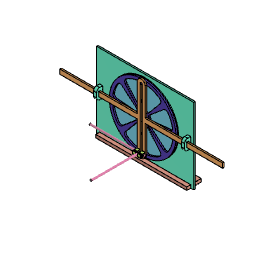
scotchYoke3D (Autodesk Fusion 360 design; units mm, degrees)
Autodesk Fusion 360 part; units mm, degrees
(part 1 of 2)
sketch "Sketch1" plane through (0, 0, 0) normal (0, 1, 0) x (1, 0, 0) in component "Wheel"
  circle A0 centre (0, 0) radius 110
  circle A1 centre (0, -100) radius 3
  line L0 (0, 0) -> (100, 0) construction
  line L1 (2.3568, -26.9387) -> (7.7954, -89.1024)
  arc A2 (6.0037, -21.6842) -> (11.0878, -19.5783) centre (0, 0) ccw
  line L2 (17.382, -20.7151) -> (57.4927, -68.5171)
  line L3 (20.7151, -17.382) -> (68.5171, -57.4927)
  line L4 (26.9387, -2.3568) -> (89.1024, -7.7954)
  arc A3 (12.5, 0) -> (1.0894, -12.4524) centre (0, 0) ccw
  arc A4 (1.0894, -12.4524) -> (8.0348, -9.5756) centre (0, 0) ccw
  arc A5 (8.0348, -9.5756) -> (9.5756, -8.0348) centre (0, 0) ccw
  arc A6 (12.4524, -1.0894) -> (12.5, 0) centre (0, 0) ccw
  arc A7 (9.5756, -8.0348) -> (12.4524, -1.0894) centre (0, 0) ccw
  arc A8 (19.7304, -98.0342) -> (55.3691, -83.2722) centre (0, 0) ccw
  arc A9 (83.2722, -55.3691) -> (98.0342, -19.7304) centre (0, 0) ccw
  arc A10 (7.7954, -89.1024) -> (19.7304, -98.0342) centre (17.7574, -88.2308) ccw
  arc A11 (55.3691, -83.2722) -> (57.4927, -68.5171) centre (49.8322, -74.945) ccw
  arc A12 (6.0037, -21.6842) -> (2.3568, -26.9387) centre (7.3378, -26.503) ccw
  arc A13 (17.382, -20.7151) -> (11.0878, -19.5783) centre (13.5518, -23.929) ccw
  arc A14 (19.5783, -11.0878) -> (20.7151, -17.382) centre (23.929, -13.5518) ccw
  arc A15 (26.9387, -2.3568) -> (21.6842, -6.0037) centre (26.503, -7.3378) ccw
  arc A16 (68.5171, -57.4927) -> (83.2722, -55.3691) centre (74.945, -49.8322) ccw
  arc A17 (98.0342, -19.7304) -> (89.1024, -7.7954) centre (88.2308, -17.7574) ccw
  arc A18 (19.7304, 98.0342) -> (7.7954, 89.1024) centre (17.7574, 88.2308) ccw
  line L5 (2.3568, 26.9387) -> (7.7954, 89.1024)
  arc A19 (2.3568, 26.9387) -> (6.0037, 21.6842) centre (7.3378, 26.503) ccw
  arc A20 (11.0878, 19.5783) -> (6.0037, 21.6842) centre (0, 0) ccw
  arc A21 (11.0878, 19.5783) -> (17.382, 20.7151) centre (13.5518, 23.929) ccw
  line L6 (17.382, 20.7151) -> (57.4927, 68.5171)
  arc A22 (57.4927, 68.5171) -> (55.3691, 83.2722) centre (49.8322, 74.945) ccw
  arc A23 (55.3691, 83.2722) -> (19.7304, 98.0342) centre (0, 0) ccw
  line L7 (20.7151, 17.382) -> (68.5171, 57.4927)
  arc A24 (83.2722, 55.3691) -> (68.5171, 57.4927) centre (74.945, 49.8322) ccw
  arc A25 (98.0342, 19.7304) -> (83.2722, 55.3691) centre (0, 0) ccw
  arc A26 (89.1024, 7.7954) -> (98.0342, 19.7304) centre (88.2308, 17.7574) ccw
  line L8 (26.9387, 2.3568) -> (89.1024, 7.7954)
  arc A27 (21.6842, 6.0037) -> (26.9387, 2.3568) centre (26.503, 7.3378) ccw
  arc A28 (21.6842, 6.0037) -> (19.5783, 11.0878) centre (0, 0) ccw
  arc A29 (20.7151, 17.382) -> (19.5783, 11.0878) centre (23.929, 13.5518) ccw
  line L9 (0, -1.75) -> (0, -22.5) construction
  arc A30 (-11.0878, -19.5783) -> (-6.0037, -21.6842) centre (0, 0) ccw
  arc A31 (-2.3568, -26.9387) -> (-6.0037, -21.6842) centre (-7.3378, -26.503) ccw
  line L10 (-2.3568, -26.9387) -> (-7.7954, -89.1024)
  line L11 (-17.382, -20.7151) -> (-57.4927, -68.5171)
  arc A32 (-19.7304, -98.0342) -> (-7.7954, -89.1024) centre (-17.7574, -88.2308) ccw
  arc A33 (-55.3691, -83.2722) -> (-19.7304, -98.0342) centre (0, 0) ccw
  arc A34 (-57.4927, -68.5171) -> (-55.3691, -83.2722) centre (-49.8322, -74.945) ccw
  arc A35 (-11.0878, -19.5783) -> (-17.382, -20.7151) centre (-13.5518, -23.929) ccw
  arc A36 (-83.2722, -55.3691) -> (-68.5171, -57.4927) centre (-74.945, -49.8322) ccw
  arc A37 (-98.0342, -19.7304) -> (-83.2722, -55.3691) centre (0, 0) ccw
  arc A38 (-89.1024, -7.7954) -> (-98.0342, -19.7304) centre (-88.2308, -17.7574) ccw
  line L12 (-26.9387, -2.3568) -> (-89.1024, -7.7954)
  arc A39 (-21.6842, -6.0037) -> (-26.9387, -2.3568) centre (-26.503, -7.3378) ccw
  arc A40 (-21.6842, -6.0037) -> (-19.5783, -11.0878) centre (0, 0) ccw
  arc A41 (-20.7151, -17.382) -> (-19.5783, -11.0878) centre (-23.929, -13.5518) ccw
  line L13 (-20.7151, -17.382) -> (-68.5171, -57.4927)
  line L14 (-20.7151, 17.382) -> (-68.5171, 57.4927)
  arc A42 (-19.5783, 11.0878) -> (-20.7151, 17.382) centre (-23.929, 13.5518) ccw
  arc A43 (-26.9387, 2.3568) -> (-21.6842, 6.0037) centre (-26.503, 7.3378) ccw
  line L15 (-26.9387, 2.3568) -> (-89.1024, 7.7954)
  arc A44 (-98.0342, 19.7304) -> (-89.1024, 7.7954) centre (-88.2308, 17.7574) ccw
  arc A45 (-83.2722, 55.3691) -> (-98.0342, 19.7304) centre (0, 0) ccw
  arc A46 (-68.5171, 57.4927) -> (-83.2722, 55.3691) centre (-74.945, 49.8322) ccw
  arc A47 (-6.0037, 21.6842) -> (-2.3568, 26.9387) centre (-7.3378, 26.503) ccw
  arc A48 (-17.382, 20.7151) -> (-11.0878, 19.5783) centre (-13.5518, 23.929) ccw
  line L16 (-17.382, 20.7151) -> (-57.4927, 68.5171)
  line L17 (-2.3568, 26.9387) -> (-7.7954, 89.1024)
  arc A49 (-7.7954, 89.1024) -> (-19.7304, 98.0342) centre (-17.7574, 88.2308) ccw
  arc A50 (-19.7304, 98.0342) -> (-55.3691, 83.2722) centre (0, 0) ccw
  arc A51 (-55.3691, 83.2722) -> (-57.4927, 68.5171) centre (-49.8322, 74.945) ccw
  arc A52 (19.5783, -11.0878) -> (21.6842, -6.0037) centre (0, 0) ccw
  arc A53 (-19.5783, 11.0878) -> (-21.6842, 6.0037) centre (0, 0) ccw
  arc A54 (-6.0037, 21.6842) -> (-11.0878, 19.5783) centre (0, 0) ccw
  dimension "d5" = 6
  dimension "d11" = 10
  dimension "d12" = 10
  dimension "d13" = 5
  dimension "d14" = 5
  dimension "d15" = 5
  dimension "d16" = 5
  dimension "d17" = 10
  dimension "d18" = 10
  constraint coincident A0.centre L0.start
  constraint horizontal L0
  constraint concentric A3 A5
  constraint concentric A4 A5
  constraint concentric A5 A6
  constraint concentric A5 A7
  constraint tangent L1 A10
  constraint tangent A8 A10
  constraint tangent L2 A11
  constraint tangent A8 A11
  constraint tangent L1 A12
  constraint tangent A2 A12
  constraint tangent L2 A13
  constraint tangent A2 A13
  constraint tangent L3 A14
  constraint tangent L4 A15
  constraint tangent L3 A16
  constraint tangent A9 A16
  constraint tangent L4 A17
  constraint tangent A9 A17
  constraint symmetric A2 L9 A30
  constraint symmetric A8 L9 A33
  constraint symmetric A9 L9 A37
  constraint symmetric L1.end L9 L10.end
  constraint symmetric A8.start L9 A32.start
  constraint symmetric A10 L9 A32
  constraint symmetric L2.end L9 L11.end
  constraint symmetric A8.end L9 A33.start
  constraint symmetric A11 L9 A34
  constraint symmetric L1.start L9 A31.start
  constraint symmetric A2.start L9 A30.end
  constraint symmetric A12 L9 A31
  constraint symmetric L2.start L9 L11.start
  constraint symmetric A2.end L9 A30.start
  constraint symmetric A13 L9 A35
  constraint symmetric L3.start L9 A41.start
  constraint symmetric A14.start L9 A40.end
  constraint symmetric A14 L9 A41
  constraint symmetric L4.start L9 L12.start
  constraint symmetric A15.end L9 A39.start
  constraint symmetric A15 L9 A39
  constraint symmetric L3.end L9 A36.end
  constraint symmetric A9.start L9 A36.start
  constraint symmetric A16 L9 A36
  constraint symmetric L4.end L9 A38.start
  constraint symmetric A9.end L9 A37.start
  constraint symmetric A17 L9 A38
  constraint symmetric A18.end L9 L17.end
  constraint symmetric A18.start L9 A49.end
  constraint symmetric A18 L9 A49
  constraint symmetric L5.start L9 A47.end
  constraint symmetric A19.end L9 A47.start
  constraint symmetric A19 L9 A47
  constraint symmetric A20.start L9 A48.end
  constraint symmetric A21.end L9 A48.start
  constraint symmetric A21 L9 A48
  constraint symmetric L6.end L9 L16.end
  constraint symmetric A22.end L9 A50.end
  constraint symmetric A22 L9 A51
  constraint symmetric A23 L9 A50
  constraint symmetric L7.start L9 L14.start
  constraint symmetric L7.end L9 L14.end
  constraint symmetric A24.start L9 A45.start
  constraint symmetric A24 L9 A46
  constraint symmetric A25.start L9 A44.start
  constraint symmetric A25 L9 A45
  constraint symmetric A26.start L9 L15.end
  constraint symmetric A26 L9 A44
  constraint symmetric L8.start L9 A43.start
  constraint symmetric A27.start L9 A43.end
  constraint symmetric A27 L9 A43
  constraint symmetric A28.end L9 A42.start
  constraint symmetric A29 L9 A42
  constraint symmetric L9 A39.start A15.end
  constraint symmetric L9 A40.end A14.start
  constraint symmetric L9 A40 A52
  measures "d5" diameter of A1
  measures "d11" radius of A10
  measures "d12" radius of A11
  measures "d13" radius of A12
  measures "d14" radius of A13
  measures "d15" radius of A14
  measures "d16" radius of A15
  measures "d17" radius of A16
  measures "d18" radius of A17
extrude "Extrude1" add sketch "Sketch1" along normal blind 5 contours A0 | A1 makes body 1 in component "Wheel"
extrude "Extrude2" add sketch "Sketch1" against normal blind 5.25 contours A1 bodies 1 in component "Wheel"
extrude "Extrude1'" add sketch "Sketch1" along normal blind 3 separate body contours A0 | A1 | L1 A2 L2 A8 A10 A11 A12 A13 | L3 L4 A9 A14 A15 A16 A17 A52 | A3 A4 A5 A6 A7 | A18 L5 A19 A20 A21 L6 A22 A23 | L7 A24 A25 A26 L8 A27 A28 A29 | A30 A31 L10 L11 A32 A33 A34 A35 | A36 A37 A38 L12 A39 A40 A41 L13 | L14 A42 A43 L15 A44 A45 A46 A53 | A47 A48 L16 L17 A49 A50 A51 A54 makes body 2 in component "BackWheel"
sketch "Sketch1 (2)" plane through (0, 0, 0) normal (0, -1, 0) x (1, 0, 0) in component "Slider"
  circle A0 centre (0, 100) radius 3
  arc A1 (26.9387, -2.3568) -> (21.6842, -6.0037) centre (26.503, -7.3378) ccw
  line L0 (26.9387, -2.3568) -> (89.1024, -7.7954)
  arc A2 (98.0342, -19.7304) -> (89.1024, -7.7954) centre (88.2308, -17.7574) ccw
  arc A3 (83.2722, -55.3691) -> (98.0342, -19.7304) centre (0, 0) ccw
  arc A4 (68.5171, -57.4927) -> (83.2722, -55.3691) centre (74.945, -49.8322) ccw
  line L1 (68.5171, -57.4927) -> (20.7151, -17.382)
  arc A5 (19.5783, -11.0878) -> (20.7151, -17.382) centre (23.929, -13.5518) ccw
  arc A6 (19.5783, -11.0878) -> (21.6842, -6.0037) centre (0, 0) ccw
  arc A7 (17.382, -20.7151) -> (11.0878, -19.5783) centre (13.5518, -23.929) ccw
  line L2 (17.382, -20.7151) -> (57.4927, -68.5171)
  arc A8 (55.3691, -83.2722) -> (57.4927, -68.5171) centre (49.8322, -74.945) ccw
  arc A9 (19.7304, -98.0342) -> (55.3691, -83.2722) centre (0, 0) ccw
  arc A10 (7.7954, -89.1024) -> (19.7304, -98.0342) centre (17.7574, -88.2308) ccw
  line L3 (7.7954, -89.1024) -> (2.3568, -26.9387)
  arc A11 (6.0037, -21.6842) -> (2.3568, -26.9387) centre (7.3378, -26.503) ccw
  arc A12 (6.0037, -21.6842) -> (11.0878, -19.5783) centre (0, 0) ccw
  circle A13 centre (0, 0) radius 12.5
  arc A14 (2.3568, 26.9387) -> (6.0037, 21.6842) centre (7.3378, 26.503) ccw
  line L4 (2.3568, 26.9387) -> (7.7954, 89.1024)
  arc A15 (19.7304, 98.0342) -> (7.7954, 89.1024) centre (17.7574, 88.2308) ccw
  arc A16 (55.3691, 83.2722) -> (19.7304, 98.0342) centre (0, 0) ccw
  arc A17 (57.4927, 68.5171) -> (55.3691, 83.2722) centre (49.8322, 74.945) ccw
  line L5 (57.4927, 68.5171) -> (17.382, 20.7151)
  arc A18 (11.0878, 19.5783) -> (17.382, 20.7151) centre (13.5518, 23.929) ccw
  arc A19 (11.0878, 19.5783) -> (6.0037, 21.6842) centre (0, 0) ccw
  line L6 (20.7151, 17.382) -> (68.5171, 57.4927)
  arc A20 (83.2722, 55.3691) -> (68.5171, 57.4927) centre (74.945, 49.8322) ccw
  arc A21 (98.0342, 19.7304) -> (83.2722, 55.3691) centre (0, 0) ccw
  arc A22 (89.1024, 7.7954) -> (98.0342, 19.7304) centre (88.2308, 17.7574) ccw
  line L7 (89.1024, 7.7954) -> (26.9387, 2.3568)
  arc A23 (21.6842, 6.0037) -> (26.9387, 2.3568) centre (26.503, 7.3378) ccw
  arc A24 (21.6842, 6.0037) -> (19.5783, 11.0878) centre (0, 0) ccw
  arc A25 (20.7151, 17.382) -> (19.5783, 11.0878) centre (23.929, 13.5518) ccw
  arc A26 (-26.9387, 2.3568) -> (-21.6842, 6.0037) centre (-26.503, 7.3378) ccw
  line L8 (-26.9387, 2.3568) -> (-89.1024, 7.7954)
  arc A27 (-98.0342, 19.7304) -> (-89.1024, 7.7954) centre (-88.2308, 17.7574) ccw
  arc A28 (-83.2722, 55.3691) -> (-98.0342, 19.7304) centre (0, 0) ccw
  arc A29 (-68.5171, 57.4927) -> (-83.2722, 55.3691) centre (-74.945, 49.8322) ccw
  line L9 (-68.5171, 57.4927) -> (-20.7151, 17.382)
  arc A30 (-19.5783, 11.0878) -> (-20.7151, 17.382) centre (-23.929, 13.5518) ccw
  arc A31 (-19.5783, 11.0878) -> (-21.6842, 6.0037) centre (0, 0) ccw
  line L10 (-2.3568, -26.9387) -> (-7.7954, -89.1024)
  arc A32 (-19.7304, -98.0342) -> (-7.7954, -89.1024) centre (-17.7574, -88.2308) ccw
  arc A33 (-55.3691, -83.2722) -> (-19.7304, -98.0342) centre (0, 0) ccw
  arc A34 (-57.4927, -68.5171) -> (-55.3691, -83.2722) centre (-49.8322, -74.945) ccw
  line L11 (-57.4927, -68.5171) -> (-17.382, -20.7151)
  arc A35 (-11.0878, -19.5783) -> (-17.382, -20.7151) centre (-13.5518, -23.929) ccw
  arc A36 (-11.0878, -19.5783) -> (-6.0037, -21.6842) centre (0, 0) ccw
  arc A37 (-2.3568, -26.9387) -> (-6.0037, -21.6842) centre (-7.3378, -26.503) ccw
  arc A38 (-6.0037, 21.6842) -> (-2.3568, 26.9387) centre (-7.3378, 26.503) ccw
  arc A39 (-6.0037, 21.6842) -> (-11.0878, 19.5783) centre (0, 0) ccw
  arc A40 (-17.382, 20.7151) -> (-11.0878, 19.5783) centre (-13.5518, 23.929) ccw
  line L12 (-17.382, 20.7151) -> (-57.4927, 68.5171)
  arc A41 (-55.3691, 83.2722) -> (-57.4927, 68.5171) centre (-49.8322, 74.945) ccw
  arc A42 (-19.7304, 98.0342) -> (-55.3691, 83.2722) centre (0, 0) ccw
  arc A43 (-7.7954, 89.1024) -> (-19.7304, 98.0342) centre (-17.7574, 88.2308) ccw
  line L13 (-7.7954, 89.1024) -> (-2.3568, 26.9387)
  line L14 (-20.7151, -17.382) -> (-68.5171, -57.4927)
  arc A44 (-83.2722, -55.3691) -> (-68.5171, -57.4927) centre (-74.945, -49.8322) ccw
  arc A45 (-98.0342, -19.7304) -> (-83.2722, -55.3691) centre (0, 0) ccw
  arc A46 (-89.1024, -7.7954) -> (-98.0342, -19.7304) centre (-88.2308, -17.7574) ccw
  line L15 (-89.1024, -7.7954) -> (-26.9387, -2.3568)
  arc A47 (-21.6842, -6.0037) -> (-26.9387, -2.3568) centre (-26.503, -7.3378) ccw
  arc A48 (-21.6842, -6.0037) -> (-19.5783, -11.0878) centre (0, 0) ccw
  arc A49 (-20.7151, -17.382) -> (-19.5783, -11.0878) centre (-23.929, -13.5518) ccw
  circle A50 centre (0, 0) radius 110
  line L16 (3.25, -100) -> (3.25, 100)
  arc A51 (3.25, 100) -> (-3.25, 100) centre (0, 100) ccw
  line L17 (-3.25, 100) -> (-3.25, -100)
  arc A52 (-3.25, -100) -> (3.25, -100) centre (0, -100) ccw
  line L18 (0, -100) -> (0, 100) construction
  line L19 (-13.25, 100) -> (-13.25, -100)
  arc A53 (-13.25, -100) -> (13.25, -100) centre (0, -100) ccw
  line L20 (13.25, -100) -> (13.25, 100)
  arc A54 (13.25, 100) -> (-13.25, 100) centre (0, 100) ccw
  dimension "d25" = 6.5
  dimension "d26" = 10
  constraint tangent L16 A51
  constraint tangent A51 L17
  constraint parallel L16 L17
  constraint tangent L17 A52
  constraint tangent L16 A52
  constraint coincident A0.centre A51.centre
  constraint vertical L18
  constraint coincident A3.centre A6.centre
  constraint midpoint L18 A3.centre
  measures "d25" diameter of A51
extrude "Extrude1''" add sketch "Sketch1 (2)" along normal blind 5 separate body contours A7 A10 L3 A11 A12 L16 L20 | A7 A11 A12 A13 A14 A18 A19 L16 L20 | A10 L3 L10 A32 A50 L16 L17 A52 L19 A53 L20 | A14 L4 A15 A18 A19 L16 L20 | L4 A15 A43 L13 A50 L16 A51 L17 L19 L20 A54 | A50 A53 | A13 L16 | A50 A54 | A13 A35 A36 A37 A38 A39 A40 L17 L19 | A13 L17 | L10 A32 A35 A36 A37 L17 L19 | A38 A39 A40 A43 L13 L17 L19 makes body 3 in component "Slider"
sketch "Sketch2" plane through (13.25, 0, 0) normal (1, 0, 0) x (0, 1, 0) in component "Slider"
  line L0 (0, -100) -> (0, 100)
  line L1 (0, 100) -> (-5, 100)
  line L2 (-5, 100) -> (-5, -100)
  line L3 (-5, -100) -> (0, -100)
  line L4 (0, 0) -> (-5, 0) construction
  line L5 (0, 7.5) -> (-5, 7.5)
  line L6 (-5, 7.5) -> (-5, -7.5)
  line L7 (-5, -7.5) -> (0, -7.5)
  line L8 (0, -7.5) -> (0, 7.5)
  line L9 (0, 7.5) -> (-5, -7.5) construction
  line L10 (-5, 7.5) -> (0, -7.5) construction
  point P0 (-2.5, 0)
  dimension "d29" = 15
  constraint coincident L4.start origin
  constraint midpoint L2 L4.end
  constraint horizontal L5
  constraint perpendicular L5 L6
  constraint parallel L5 L7
  constraint parallel L6 L8
  constraint coincident L9 P0
  constraint coincident L10 P0
  constraint midpoint L4 P0
  measures "d29" distance of L5.end L6.end
extrude "Extrude2'" add sketch "Sketch2" along normal blind 255 contours L0 L2 L5 L6 L7 L8 bodies 3 in component "Slider"
mirror "Mirror1" about plane through (0, 0, 0) normal (1, 0, 0) of "Extrude2'" in component "Slider"
sketch "Sketch1 (3)" plane through (0, 8, 0) normal (0, 1, 0) x (-1, 0, 0) in component "Board"
  circle A0 centre (0, 0) radius 110
  line L0 (-120, 120) -> (120, 120) construction
  line L1 (120, 120) -> (120, -120) construction
  line L2 (120, -120) -> (-120, -120) construction
  line L3 (-120, -120) -> (-120, 120) construction
  line L4 (-120, 120) -> (120, -120) construction
  line L5 (120, 120) -> (-120, -120) construction
  line L6 (120, 0) -> (130, 0) construction
  line L7 (-120, 0) -> (-130, 0) construction
  line L8 (0, -120) -> (0, -130) construction
  circle A1 centre (0, 0) radius 12.5
  line L9 (0, 0) -> (-150, 0) construction
  line L10 (0, 0) -> (150, 0) construction
  line L11 (150, -130) -> (160, -130) construction
  line L12 (-150, -130) -> (-160, -130) construction
  line L13 (-150, 120) -> (-160, 120) construction
  line L14 (150, 120) -> (160, 120) construction
  line L15 (160, -130) -> (-160, -130)
  line L16 (-160, -130) -> (-160, 120)
  line L17 (-160, 120) -> (160, 120)
  line L18 (160, 120) -> (160, -130)
  dimension "d34" = 240
  dimension "d35" = 240
  dimension "d39" = 25
  dimension "d72" = 150
  dimension "d255" = 10
  dimension "d256" = 10
  dimension "d257" = 10
  dimension "d258" = 10
  constraint horizontal L0
  constraint perpendicular L0 L1
  constraint parallel L0 L2
  constraint parallel L1 L3
  constraint coincident L4 A0.centre
  constraint coincident L5 A0.centre
  constraint coincident A0.centre A1.centre
  constraint midpoint L1 L6.start
  constraint perpendicular L1 L6
  constraint midpoint L3 L7.start
  constraint perpendicular L3 L7
  constraint midpoint L2 L8.start
  constraint perpendicular L2 L8
  constraint horizontal L9
  constraint horizontal L15
  constraint vertical L16
  constraint horizontal L17
  constraint vertical L18
  measures "d34" distance of L1.end L2.end
  measures "d35" distance of L0.end L1.end
  measures "d39" diameter of A1
  measures "d72" distance of A0.centre L9.end
  measures "d255" distance of L11.start L11.end
  measures "d256" distance of L12.start L12.end
  measures "d257" distance of L13.start L13.end
  measures "d258" distance of L14.start L14.end
extrude "Extrude1'''" add sketch "Sketch1 (3)" along normal blind 5 separate body contours A0 | L15 L16 L17 L18 makes body 4 in component "Board"
sketch "Sketch2 (2)" plane through (0, 8, 0) normal (0, -1, 0) x (1, 0, 0) in component "Board"
  circle A0 centre (0, 0) radius 12.5
  line L0 (-130, -130) -> (130, -130) construction
  line L1 (-120, -130) -> (-80, -130)
  line L2 (-80, -130) -> (-80, -120)
  line L3 (-80, -120) -> (-120, -120)
  line L4 (-120, -120) -> (-120, -130)
  line L5 (-70, -130) -> (-30, -130)
  line L6 (-30, -130) -> (-30, -120)
  line L7 (-30, -120) -> (-70, -120)
  line L8 (-70, -120) -> (-70, -130)
  line L9 (-20, -130) -> (20, -130)
  line L10 (20, -130) -> (20, -120)
  line L11 (20, -120) -> (-20, -120)
  line L12 (-20, -120) -> (-20, -130)
  line L13 (30, -130) -> (70, -130)
  line L14 (70, -130) -> (70, -120)
  line L15 (70, -120) -> (30, -120)
  line L16 (30, -120) -> (30, -130)
  line L17 (80, -130) -> (120, -130)
  line L18 (120, -130) -> (120, -120)
  line L19 (120, -120) -> (80, -120)
  line L20 (80, -120) -> (80, -130)
  line L21 (130, -130) -> (150, -130)
  line L22 (150, -130) -> (150, -120)
  line L23 (150, -120) -> (130, -120)
  line L24 (130, -120) -> (130, -130)
  line L25 (-130, -130) -> (-150, -130)
  line L26 (-150, -130) -> (-150, -120)
  line L27 (-150, -120) -> (-130, -120)
  line L28 (-130, -120) -> (-130, -130)
  line L29 (160, 120) -> (-160, 120)
  line L30 (-160, 120) -> (-160, -130)
  line L31 (-160, -130) -> (160, -130)
  line L32 (160, -130) -> (160, 120)
  dimension "d42" = 40
  dimension "d43" = 10
  dimension "d45" = 40
  dimension "d46" = 10
  dimension "d47" = 10
  dimension "d48" = 40
  dimension "d49" = 10
  dimension "d50" = 40
  dimension "d51" = 10
  dimension "d52" = 10
  dimension "d53" = 40
  dimension "d54" = 10
  dimension "d55" = 10
  constraint horizontal L1
  constraint vertical L2
  constraint horizontal L3
  constraint vertical L4
  constraint coincident L0 L1.start
  constraint horizontal L5
  constraint vertical L6
  constraint horizontal L7
  constraint vertical L8
  constraint coincident L0 L5.start
  constraint horizontal L9
  constraint vertical L10
  constraint horizontal L11
  constraint vertical L12
  constraint coincident L0 L9.start
  constraint horizontal L13
  constraint vertical L14
  constraint horizontal L15
  constraint vertical L16
  constraint coincident L0 L13.start
  constraint horizontal L17
  constraint vertical L18
  constraint horizontal L19
  constraint vertical L20
  constraint coincident L0 L17.start
  constraint horizontal L21
  constraint vertical L22
  constraint horizontal L23
  constraint vertical L24
  constraint horizontal L25
  constraint vertical L26
  constraint horizontal L27
  constraint vertical L28
  measures "d42" distance of L1.start L1.end
  measures "d43" distance of L1.start L3.end
  measures "d45" distance of L5.start L5.end
  measures "d46" distance of L5.start L7.end
  measures "d47" distance of L2 L8
  measures "d48" distance of L9.start L9.end
  measures "d49" distance of L6 L12
  measures "d50" distance of L13.start L13.end
  measures "d51" distance of L13.start L15.end
  measures "d52" distance of L10 L16
  measures "d53" distance of L17.start L17.end
  measures "d54" distance of L17.start L19.end
  measures "d55" distance of L14 L20
extrude "Extrude2''" cut sketch "Sketch2 (2)" against normal blind 5 contours L1 L2 L3 L4 L31 | L25 L26 L27 L28 L31 | L5 L6 L7 L8 L31 | L9 L10 L11 L12 L31 | L13 L14 L15 L16 L31 | L21 L22 L23 L24 L31 | L17 L18 L19 L20 L31 bodies 4 in component "Board"
sketch "Sketch1 (4)" plane through (0, 8, 0) normal (0, -1, 0) x (1, 0, 0) in component "Base"
  line L0 (-20, -130) -> (-20, -120)
  line L1 (-20, -120) -> (20, -120)
  line L2 (20, -120) -> (20, -130)
  line L3 (30, -130) -> (30, -120)
  line L4 (30, -120) -> (70, -120)
  line L5 (70, -120) -> (70, -130)
  line L6 (80, -130) -> (80, -120)
  line L7 (80, -120) -> (120, -120)
  line L8 (120, -120) -> (120, -130)
  line L9 (-120, -130) -> (-120, -120)
  line L10 (-120, -120) -> (-80, -120)
  line L11 (-80, -120) -> (-80, -130)
  line L12 (-70, -130) -> (-70, -120)
  line L13 (-70, -120) -> (-30, -120)
  line L14 (-30, -120) -> (-30, -130)
  circle A0 centre (0, 0) radius 12.5
  line L15 (-130, -130) -> (130, -130)
  line L16 (130, -130) -> (130, -120)
  line L17 (130, -120) -> (-130, -120)
  line L18 (-130, -120) -> (-130, -130)
  line L19 (130, -130) -> (130, -120)
  line L20 (130, -120) -> (150, -120)
  line L21 (-150, -120) -> (-130, -120)
  line L22 (-130, -120) -> (-130, -130)
  line L23 (120, -130) -> (130, -130)
  line L24 (150, -120) -> (150, -130)
  line L25 (150, -130) -> (160, -130)
  line L26 (160, -130) -> (160, 120)
  line L27 (160, 120) -> (-160, 120)
  line L28 (-160, 120) -> (-160, -130)
  line L29 (-160, -130) -> (-150, -130)
  line L30 (-150, -130) -> (-150, -120)
  line L31 (-130, -130) -> (-120, -130)
  line L32 (-80, -130) -> (-70, -130)
  line L33 (-30, -130) -> (-20, -130)
  line L34 (20, -130) -> (30, -130)
  line L35 (70, -130) -> (80, -130)
  constraint horizontal L15
  constraint vertical L16
  constraint horizontal L17
  constraint vertical L18
extrude "Extrude1''''" add sketch "Sketch1 (4)" along normal blind 13 separate body contours L0 L14 L15 L17 L33 | L0 L1 L2 L15 L17 | L12 L13 L14 L15 L17 | L2 L3 L15 L17 L34 | L11 L12 L15 L17 L32 | L3 L4 L5 L15 L17 | L9 L10 L11 L15 L17 | L5 L6 L15 L17 L35 | L9 L15 L17 L18 L22 L31 | L6 L7 L8 L15 L17 | L8 L15 L16 L17 L19 L23 makes body 5 in component "Base"
sketch "Sketch2 (3)" plane through (0, 8, 0) normal (0, 1, 0) x (-1, 0, 0) in component "Base"
  line L0 (130, -130) -> (130, -120)
  line L1 (130, -120) -> (-130, -120)
  line L2 (-130, -120) -> (-130, -130)
  line L3 (-130, -130) -> (130, -130)
  line L4 (-130, -130) -> (130, -130)
  line L5 (130, -130) -> (130, -120)
  line L6 (130, -120) -> (-130, -120)
  line L7 (-130, -120) -> (-130, -130)
  line L8 (-120, -130) -> (-80, -130)
  line L9 (-80, -130) -> (-80, -120)
  line L10 (-80, -120) -> (-120, -120)
  line L11 (-120, -120) -> (-120, -130)
  line L12 (-70, -130) -> (-30, -130)
  line L13 (-30, -130) -> (-30, -120)
  line L14 (-30, -120) -> (-70, -120)
  line L15 (-70, -120) -> (-70, -130)
  line L16 (-20, -130) -> (20, -130)
  line L17 (20, -130) -> (20, -120)
  line L18 (20, -120) -> (-20, -120)
  line L19 (-20, -120) -> (-20, -130)
  line L20 (30, -130) -> (70, -130)
  line L21 (70, -130) -> (70, -120)
  line L22 (70, -120) -> (30, -120)
  line L23 (30, -120) -> (30, -130)
  line L24 (80, -130) -> (120, -130)
  line L25 (120, -130) -> (120, -120)
  line L26 (120, -120) -> (80, -120)
  line L27 (80, -120) -> (80, -130)
  constraint horizontal L4
  constraint vertical L5
  constraint horizontal L6
  constraint vertical L7
  constraint coincident L0.end L1.start
  constraint coincident L2.end L3.start
  constraint horizontal L8
  constraint vertical L9
  constraint horizontal L10
  constraint vertical L11
  constraint coincident L6 L9.end
  constraint horizontal L12
  constraint vertical L13
  constraint horizontal L14
  constraint vertical L15
  constraint coincident L6 L13.end
  constraint coincident L4 L12.start
  constraint horizontal L16
  constraint vertical L17
  constraint horizontal L18
  constraint vertical L19
  constraint coincident L6 L17.end
  constraint coincident L4 L16.start
  constraint horizontal L20
  constraint vertical L21
  constraint horizontal L22
  constraint vertical L23
  constraint coincident L6 L21.end
  constraint coincident L4 L20.start
  constraint horizontal L24
  constraint vertical L25
  constraint horizontal L26
  constraint vertical L27
  constraint coincident L6 L25.end
  constraint coincident L4 L24.start
extrude "Extrude2'''" add sketch "Sketch2 (3)" along normal blind 5 contours L1 L3 L4 L6 L24 L25 L26 L27 | L1 L3 L4 L6 L20 L21 L22 L23 | L1 L3 L4 L6 L16 L17 L18 L19 | L1 L3 L4 L6 L12 L13 L14 L15 | L1 L3 L4 L6 L8 L9 L10 L11 bodies 5 in component "Base"
sketch "Sketch3" plane through (0, 13, 0) normal (0, 1, 0) x (-1, 0, 0) in component "Base"
  line L0 (-120, -120) -> (-120, -130)
  line L1 (-120, -130) -> (-80, -130)
  line L2 (-80, -130) -> (-80, -120)
  line L3 (-80, -120) -> (-120, -120)
  line L4 (-130, -130) -> (130, -130)
  line L5 (130, -130) -> (130, -120)
  line L6 (130, -120) -> (-130, -120)
  line L7 (-130, -120) -> (-130, -130)
  constraint horizontal L4
  constraint vertical L5
  constraint horizontal L6
  constraint vertical L7
extrude "Extrude3" add sketch "Sketch3" along normal blind 30 bodies 5 in component "Base"
sketch "Sketch4" plane through (-130, 0, 0) normal (-1, 0, 0) x (0, -1, 0) in component "Base"
  line L0 (-13, -130) -> (-13, -120)
  line L1 (-13, -120) -> (-43, -120)
  line L2 (-43, -120) -> (-43, -130)
  line L3 (-43, -130) -> (-13, -130)
  line L4 (-43, -130) -> (5, -130)
  line L5 (5, -130) -> (5, -120)
  line L6 (5, -120) -> (-43, -120)
  line L7 (-43, -120) -> (-43, -130)
  dimension "d64" = 48
  dimension "d65" = 10
  constraint horizontal L4
  constraint vertical L5
  constraint horizontal L6
  constraint vertical L7
  constraint coincident L2.end L3.start
  measures "d64" distance of L2.end L4.end
  measures "d65" distance of L2.end L1.end
extrude "Extrude4" add sketch "Sketch4" along normal blind 20 bodies 5 in component "Base"
sketch "Sketch5" plane through (130, 0, 0) normal (1, 0, 0) x (0, 1, 0) in component "Base"
  line L0 (13, -120) -> (13, -130)
  line L1 (13, -130) -> (43, -130)
  line L2 (43, -130) -> (43, -120)
  line L3 (43, -120) -> (13, -120)
  line L4 (43, -130) -> (-5, -130)
  line L5 (-5, -130) -> (-5, -120)
  line L6 (-5, -120) -> (43, -120)
  line L7 (43, -120) -> (43, -130)
  dimension "d68" = 48
  dimension "d69" = 10
  constraint horizontal L4
  constraint vertical L5
  constraint horizontal L6
  constraint vertical L7
  constraint coincident L1.end L2.start
  measures "d68" distance of L1.end L4.end
  measures "d69" distance of L1.end L2.end
extrude "Extrude5" add sketch "Sketch5" along normal blind 20 bodies 5 in component "Base"
sketch "Sketch4 (2)" plane through (0, 8, 0) normal (0, -1, 0) x (1, 0, 0) in component "Board"
  circle A0 centre (0, 0) radius 12.5
  line L0 (80, -130) -> (80, -120)
  line L1 (80, -120) -> (120, -120)
  line L2 (120, -120) -> (120, -130)
  line L3 (130, -130) -> (130, -120)
  line L4 (130, -120) -> (150, -120)
  line L5 (-150, -120) -> (-130, -120)
  line L6 (-130, -120) -> (-130, -130)
  line L7 (-120, -130) -> (-120, -120)
  line L8 (-120, -120) -> (-80, -120)
  line L9 (-80, -120) -> (-80, -130)
  line L10 (-70, -130) -> (-70, -120)
  line L11 (-70, -120) -> (-30, -120)
  line L12 (-30, -120) -> (-30, -130)
  line L13 (-20, -130) -> (-20, -120)
  line L14 (-20, -120) -> (20, -120)
  line L15 (20, -120) -> (20, -130)
  line L16 (30, -130) -> (30, -120)
  line L17 (30, -120) -> (70, -120)
  line L18 (70, -120) -> (70, -130)
  line L19 (150, 0) -> (140, 0) construction
  line L20 (150, 17.5) -> (140, 17.5)
  line L21 (140, 17.5) -> (140, -17.5)
  line L22 (140, -17.5) -> (150, -17.5)
  line L23 (150, -17.5) -> (150, 17.5)
  line L24 (150, 17.5) -> (140, -17.5) construction
  line L25 (140, 17.5) -> (150, -17.5) construction
  line L26 (0, 1.75) -> (0, 22.5)
  line L27 (-140, 17.5) -> (-140, -17.5)
  line L28 (-150, 17.5) -> (-140, 17.5)
  line L29 (-150, -17.5) -> (-150, 17.5)
  line L30 (-140, -17.5) -> (-150, -17.5)
  line L31 (120, -130) -> (130, -130)
  line L32 (150, -120) -> (150, -130)
  line L33 (150, -130) -> (160, -130)
  line L34 (160, -130) -> (160, 120)
  line L35 (160, 120) -> (-160, 120)
  line L36 (-160, 120) -> (-160, -130)
  line L37 (-160, -130) -> (-150, -130)
  line L38 (-150, -130) -> (-150, -120)
  line L39 (-130, -130) -> (-120, -130)
  line L40 (-80, -130) -> (-70, -130)
  line L41 (-30, -130) -> (-20, -130)
  line L42 (20, -130) -> (30, -130)
  line L43 (70, -130) -> (80, -130)
  point P0 (145, 0)
  dimension "d73" = 35
  constraint horizontal L20
  constraint perpendicular L20 L21
  constraint parallel L20 L22
  constraint parallel L21 L23
  constraint coincident L24 P0
  constraint coincident L25 P0
  constraint midpoint L19 P0
  constraint symmetric L20.start L26 L28.start
  constraint symmetric L20.end L26 L27.start
  constraint symmetric L21.end L26 L27.end
  constraint symmetric L22.end L26 L29.start
  measures "d73" distance of L20.end L21.end
extrude "Extrude3'" add sketch "Sketch4 (2)" along normal blind 20 separate body contours L20 L21 L22 L23 | L27 L28 L29 L30 makes body 6 at (-140, 1.3333, 5.8333) makes body 7 at (150, 1.3333, -5.8333) in component "Board"
sketch "Sketch5 (2)" plane through (150, 0, 0) normal (1, 0, 0) x (0, 1, 0) in component "Board"
  line L0 (8, 17.5) -> (-12, 17.5)
  line L1 (-12, 17.5) -> (-12, -17.5)
  line L2 (-12, -17.5) -> (8, -17.5)
  line L3 (0, 0) -> (-5, 0) construction
  line L4 (0.25, 7.75) -> (-5.25, 7.75)
  line L5 (-5.25, 7.75) -> (-5.25, -7.75)
  line L6 (-5.25, -7.75) -> (0.25, -7.75)
  line L7 (0.25, -7.75) -> (0.25, 7.75)
  line L8 (0.25, 7.75) -> (-5.25, -7.75) construction
  line L9 (-5.25, 7.75) -> (0.25, -7.75) construction
  line L10 (8, -17.5) -> (8, 17.5)
  point P0 (-2.5, 0)
  dimension "d76" = 5.5
  dimension "d77" = 15.5
  constraint coincident L3.start origin
  constraint horizontal L3
  constraint horizontal L4
  constraint perpendicular L4 L5
  constraint parallel L4 L6
  constraint parallel L5 L7
  constraint coincident L8 P0
  constraint coincident L9 P0
  constraint midpoint L3 P0
  measures "d76" distance of L5.end L6.end
  measures "d77" distance of L4.end L5.end
extrude "Extrude4'" cut sketch "Sketch5 (2)" against normal blind 325 contours L4 L5 L6 L7 bodies 7 6 4 in component "Board"
sketch "Sketch6" plane through (150, 0, 0) normal (1, 0, 0) x (0, 1, 0) in component "Board"
  line L0 (-5.25, 7.75) -> (0.25, 7.75)
  line L1 (0.25, 7.75) -> (0.25, -7.75)
  line L2 (0.25, -7.75) -> (-5.25, -7.75)
  line L3 (-5.25, -7.75) -> (-5.25, 7.75)
  line L4 (8, 17.5) -> (-12, 17.5)
  line L5 (-12, 17.5) -> (-12, -17.5)
  line L6 (-12, -17.5) -> (8, -17.5)
  line L7 (-2, 17.5) -> (8, 17.5)
  line L8 (8, 17.5) -> (8, -17.5)
  line L9 (8, -17.5) -> (-2, -17.5)
  line L10 (-12, -7.5) -> (-12, 7.5)
  arc A0 (-2, 17.5) -> (-12, 7.5) centre (-2, 7.5) ccw
  arc A1 (-12, -7.5) -> (-2, -17.5) centre (-2, -7.5) ccw
  line L11 (8, -17.5) -> (8, 17.5)
  dimension "d80" = 10
  dimension "d81" = 10
  constraint horizontal L7
  constraint vertical L8
  constraint horizontal L9
  constraint vertical L10
  constraint coincident L6.end L8.end
  constraint tangent L7 A0
  constraint tangent L10 A0
  constraint tangent L10 A1
  constraint tangent L9 A1
  measures "d80" radius of A0
  measures "d81" radius of A1
extrude "Extrude5'" cut sketch "Sketch6" against normal blind 310 contours L4 L5 A0 | L5 L6 A1 bodies 7 4 6 in component "Board"
sketch "Sketch2 (4)" plane through (0, 3, 0) normal (0, 1, 0) x (-1, 0, 0) in component "BackWheel"
  circle A0 centre (0, 0) radius 110
  circle A1 centre (0, 0) radius 12.5
  dimension "d136" = 25
  constraint coincident A0.centre A1.centre
  measures "d136" diameter of A1
extrude "Extrude2''''" add sketch "Sketch2 (4)" along normal blind 5 contours A1 bodies 2 in component "BackWheel"
move_body "Align5" bodies 3 to x (1, 0, 0) y (0, 1, 0) z (0, 0, 1) at (1.75, 0, 0.25) in component "Slider"
move_body "Align6" bodies 3 to x (1, 0, 0) y (0, 1, 0) z (0, 0, 1) at (0, 0, 0) in component "Slider"
sketch "Sketch2 (5)" plane through (0, -5, 0) normal (0, -1, 0) x (1, 0, 0) in component "HangerBase"
  arc A0 (-3.25, -100) -> (3.25, -100) centre (0, -100) ccw
  line L0 (-3.25, -100) -> (-3.25, 100)
  arc A1 (3.25, 100) -> (-3.25, 100) centre (0, 100) ccw
  line L1 (3.25, 100) -> (3.25, -100)
  arc A2 (13.25, 100) -> (-13.25, 100) centre (0, 100) ccw
  line L2 (-13.25, 100) -> (-13.25, 7.5)
  line L3 (-13.25, 7.5) -> (-268.25, 7.5)
  line L4 (-268.25, 7.5) -> (-268.25, -7.5)
  line L5 (-268.25, -7.5) -> (-13.25, -7.5)
  line L6 (-13.25, -7.5) -> (-13.25, -100)
  arc A3 (-13.25, -100) -> (13.25, -100) centre (0, -100) ccw
  line L7 (13.25, -100) -> (13.25, -7.5)
  line L8 (13.25, -7.5) -> (268.25, -7.5)
  line L9 (268.25, -7.5) -> (268.25, 7.5)
  line L10 (268.25, 7.5) -> (13.25, 7.5)
  line L11 (13.25, 7.5) -> (13.25, 100)
  line L12 (-13.25, -100) -> (-3.25, -100)
  line L13 (-3.25, -100) -> (-3.25, -90)
  line L14 (-3.25, -90) -> (-13.25, -90)
  line L15 (-13.25, -90) -> (-13.25, -100)
  line L16 (3.25, -100) -> (13.25, -100)
  line L17 (13.25, -100) -> (13.25, -90)
  line L18 (13.25, -90) -> (3.25, -90)
  line L19 (3.25, -90) -> (3.25, -100)
  dimension "d167" = 10
  dimension "d168" = 10
  dimension "d169" = 10
  dimension "d170" = 10
  constraint horizontal L12
  constraint vertical L13
  constraint horizontal L14
  constraint vertical L15
  constraint coincident L6.end A3.start
  constraint horizontal L16
  constraint vertical L17
  constraint horizontal L18
  constraint vertical L19
  constraint coincident A0.end L1.end
  measures "d167" distance of L6.end A0.start
  measures "d168" distance of L6.end L14.end
  measures "d169" distance of A0.end A3.end
  measures "d170" distance of A0.end L18.end
extrude "Extrude1'''''" add sketch "Sketch2 (5)" along normal blind 15.2 separate body contours L0 L6 L12 L13 L14 L15 | L1 L7 L16 L17 L18 L19 makes body 8 at (-9.9167, -15.1333, -100) makes body 9 at (3.25, -15.1333, -93.3333) in component "HangerBase"
sketch "Sketch3 (2)" plane through (13.25, 0, 0) normal (1, 0, 0) x (0, 1, 0) in component "HangerBase"
  line L0 (-5, -100) -> (-5, -90)
  line L1 (-5, -90) -> (-20.2, -90)
  line L2 (-20.2, -90) -> (-20.2, -100)
  line L3 (-20.2, -100) -> (-5, -100)
  line L4 (-5, -95) -> (-10.05, -95) construction
  circle A0 centre (-10.05, -95) radius 3.05
  line L5 (-20.2, -95) -> (-16.65, -95) construction
  line L6 (-16.65, -100) -> (-16.65, -98) construction
  line L7 (-16.65, -98) -> (-16.65, -90) construction
  line L8 (-15.1, -90) -> (-18.2, -90)
  line L9 (-18.2, -90) -> (-18.2, -98)
  line L10 (-18.2, -98) -> (-15.1, -98)
  line L11 (-15.1, -98) -> (-15.1, -90)
  line L12 (-15.1, -90) -> (-18.2, -98) construction
  line L13 (-18.2, -90) -> (-15.1, -98) construction
  point P0 (-16.65, -94)
  dimension "d173" = 5.05
  dimension "d174" = 6.1
  dimension "d175" = 3.55
  dimension "d176" = 2
  dimension "d177" = 3.1
  dimension "d178" = 8
  constraint midpoint L0 L4.start
  constraint perpendicular L0 L4
  constraint coincident L4.end A0.centre
  constraint midpoint L2 L5.start
  constraint perpendicular L2 L5
  constraint vertical L6
  constraint coincident L3 L6.start
  constraint coincident L1 L7.end
  constraint perpendicular L1 L7
  constraint horizontal L8
  constraint perpendicular L8 L9
  constraint parallel L8 L10
  constraint parallel L9 L11
  constraint coincident L12 P0
  constraint coincident L13 P0
  constraint midpoint L7 P0
  measures "d173" distance of L4.start L4.end
  measures "d174" diameter of A0
  measures "d175" distance of L5.start L5.end
  measures "d176" distance of L6.start L6.end
  measures "d177" distance of L9.end L10.end
  measures "d178" distance of L8.end L9.end
extrude "Extrude2'''''" cut sketch "Sketch3 (2)" against normal blind 31 contours L1 L8 L9 L10 L11 | A0 bodies 8 9 in component "HangerBase"
sketch "Sketch1 (5)" plane through (13.25, 0, 0) normal (1, 0, 0) x (0, 1, 0) in component "HangerSideways"
  line L0 (-15.1, -90) -> (-15.1, -98)
  line L1 (-15.1, -98) -> (-18.2, -98)
  line L2 (-18.2, -98) -> (-18.2, -90)
  line L3 (-18.2, -90) -> (-20.2, -90)
  line L4 (-20.2, -90) -> (-20.2, -100)
  line L5 (-20.2, -100) -> (-5, -100)
  line L6 (-5, -100) -> (-5, -90)
  line L7 (-5, -90) -> (-15.1, -90)
  circle A0 centre (-10.05, -95) radius 3.05
  circle A1 centre (-10.05, -95) radius 4.5
  dimension "d181" = 9
  constraint concentric A0 A1
  measures "d181" diameter of A1
extrude "Extrude1''''''" add sketch "Sketch1 (5)" along normal blind 3 separate body contours A0 | A1 makes body 10 in component "HangerSideways"
sketch "Sketch2 (6)" plane through (13.25, 0, 0) normal (-1, 0, 0) x (0, -1, 0) in component "HangerSideways"
  circle A0 centre (10.05, -95) radius 4.5
  circle A1 centre (10.05, -95) radius 3
  dimension "d184" = 6
  constraint concentric A0 A1
  measures "d184" diameter of A1
extrude "Extrude2''''''" add sketch "Sketch2 (6)" along normal blind 176.5 contours A1 bodies 10 in component "HangerSideways"
sketch "Sketch1 (6)" plane through (0, -15.1, 0) normal (0, -1, 0) x (1, 0, 0) in component "HangerOutin"
  line L0 (3.25, -90) -> (3.25, -98)
  line L1 (3.25, -98) -> (13.25, -98)
  line L2 (13.25, -98) -> (13.25, -90)
  line L3 (13.25, -90) -> (3.25, -90)
  line L4 (13.25, -90) -> (-13.25, -90)
  line L5 (-13.25, -90) -> (-13.25, -98)
  line L6 (-13.25, -98) -> (13.25, -98)
  line L7 (13.25, -98) -> (13.25, -90)
  dimension "d192" = 26.5
  constraint horizontal L4
  constraint vertical L5
  constraint horizontal L6
  constraint vertical L7
  constraint coincident L2.end L3.start
  measures "d192" distance of L2.end L4.end
extrude "Extrude1'''''''" add sketch "Sketch1 (6)" along normal blind 3 separate body makes body 11 in component "HangerOutin"
sketch "Sketch2 (7)" plane through (0, -18.1, 0) normal (0, -1, 0) x (1, 0, 0) in component "HangerOutin"
  line L0 (13.25, -98) -> (13.25, -90)
  line L1 (13.25, -90) -> (-13.25, -90)
  line L2 (-13.25, -90) -> (-13.25, -98)
  line L3 (-13.25, -98) -> (13.25, -98)
  circle A0 centre (0, -94) radius 3
  dimension "d195" = 6
  measures "d195" diameter of A0
extrude "Extrude2'''''''" add sketch "Sketch2 (7)" along normal blind 152 contours A0 bodies 11 in component "HangerOutin"
sketch "Sketch4 (3)" plane through (0, 0, 0) normal (0, -1, 0) x (1, 0, 0) in component "BackWheel"
  circle A0 centre (0, 0) radius 110
  circle A1 centre (0, 0) radius 110
  circle A2 centre (0, 0) radius 12.7
  circle A3 centre (0, 0) radius 9.5 construction
  line L0 (0, 0) -> (9.5, 0) construction
  line L1 (0, 0) -> (0, 9.5) construction
  line L2 (0, 0) -> (4.75, 8.2272) construction
  line L3 (0, 0) -> (9.5, 0) construction
  line L4 (0, 0) -> (4.75, -8.2272) construction
  circle A4 centre (9.5, 0) radius 1.5
  circle A5 centre (4.75, 8.2272) radius 1.5
  circle A6 centre (4.75, -8.2272) radius 1.5
  circle A7 centre (-4.75, 8.2272) radius 1.5
  circle A8 centre (-9.5, 0) radius 1.5
  circle A9 centre (-4.75, -8.2272) radius 1.5
  dimension "d242" = 25.4
  dimension "d243" = 19
  dimension "d244" = 60
  dimension "d245" = 60
  dimension "d246" = 3
  dimension "d247" = 3
  dimension "d248" = 3
  constraint coincident A0.centre A1.centre
  constraint concentric A1 A2
  constraint concentric A2 A3
  constraint coincident A3 L0.end
  constraint horizontal L0
  constraint coincident A3 L1.end
  constraint vertical L1
  constraint horizontal L3
  constraint coincident A3 L2.end
  constraint coincident A3 L4.end
  constraint coincident L0.end L3.end
  constraint coincident L2.end A5.centre
  constraint coincident L4.end A6.centre
  constraint symmetric L1 A4 A8
  constraint symmetric L1 A5 A7
  constraint symmetric L1 A6 A9
  measures "d242" diameter of A2
  measures "d243" diameter of A3
  measures "d244" angle of L2 L3
  measures "d245" angle of L2 L4
  measures "d246" diameter of A4
  measures "d247" diameter of A5
  measures "d248" diameter of A6
extrude "Extrude3''" cut sketch "Sketch4 (3)" against normal blind 8 contours A4 | A5 | A6 | A7 | A8 | A9 bodies 2 in component "BackWheel"
sketch "Sketch2 (8)" plane through (0, 0, 0) normal (0, -1, 0) x (1, 0, 0) in component "Wheel"
  circle A0 centre (0, 100) radius 3
  arc A1 (26.9387, -2.3568) -> (21.6842, -6.0037) centre (26.503, -7.3378) ccw
  line L0 (26.9387, -2.3568) -> (89.1024, -7.7954)
  arc A2 (98.0342, -19.7304) -> (89.1024, -7.7954) centre (88.2308, -17.7574) ccw
  arc A3 (83.2722, -55.3691) -> (98.0342, -19.7304) centre (0, 0) ccw
  arc A4 (68.5171, -57.4927) -> (83.2722, -55.3691) centre (74.945, -49.8322) ccw
  line L1 (68.5171, -57.4927) -> (20.7151, -17.382)
  arc A5 (19.5783, -11.0878) -> (20.7151, -17.382) centre (23.929, -13.5518) ccw
  arc A6 (19.5783, -11.0878) -> (21.6842, -6.0037) centre (0, 0) ccw
  arc A7 (17.382, -20.7151) -> (11.0878, -19.5783) centre (13.5518, -23.929) ccw
  line L2 (17.382, -20.7151) -> (57.4927, -68.5171)
  arc A8 (55.3691, -83.2722) -> (57.4927, -68.5171) centre (49.8322, -74.945) ccw
  arc A9 (19.7304, -98.0342) -> (55.3691, -83.2722) centre (0, 0) ccw
  arc A10 (7.7954, -89.1024) -> (19.7304, -98.0342) centre (17.7574, -88.2308) ccw
  line L3 (7.7954, -89.1024) -> (2.3568, -26.9387)
  arc A11 (6.0037, -21.6842) -> (2.3568, -26.9387) centre (7.3378, -26.503) ccw
  arc A12 (6.0037, -21.6842) -> (11.0878, -19.5783) centre (0, 0) ccw
  circle A13 centre (0, 0) radius 12.5
  arc A14 (2.3568, 26.9387) -> (6.0037, 21.6842) centre (7.3378, 26.503) ccw
  line L4 (2.3568, 26.9387) -> (7.7954, 89.1024)
  arc A15 (19.7304, 98.0342) -> (7.7954, 89.1024) centre (17.7574, 88.2308) ccw
  arc A16 (55.3691, 83.2722) -> (19.7304, 98.0342) centre (0, 0) ccw
  arc A17 (57.4927, 68.5171) -> (55.3691, 83.2722) centre (49.8322, 74.945) ccw
  line L5 (57.4927, 68.5171) -> (17.382, 20.7151)
  arc A18 (11.0878, 19.5783) -> (17.382, 20.7151) centre (13.5518, 23.929) ccw
  arc A19 (11.0878, 19.5783) -> (6.0037, 21.6842) centre (0, 0) ccw
  line L6 (20.7151, 17.382) -> (68.5171, 57.4927)
  arc A20 (83.2722, 55.3691) -> (68.5171, 57.4927) centre (74.945, 49.8322) ccw
  arc A21 (98.0342, 19.7304) -> (83.2722, 55.3691) centre (0, 0) ccw
  arc A22 (89.1024, 7.7954) -> (98.0342, 19.7304) centre (88.2308, 17.7574) ccw
  line L7 (89.1024, 7.7954) -> (26.9387, 2.3568)
  arc A23 (21.6842, 6.0037) -> (26.9387, 2.3568) centre (26.503, 7.3378) ccw
  arc A24 (21.6842, 6.0037) -> (19.5783, 11.0878) centre (0, 0) ccw
  arc A25 (20.7151, 17.382) -> (19.5783, 11.0878) centre (23.929, 13.5518) ccw
  arc A26 (-26.9387, 2.3568) -> (-21.6842, 6.0037) centre (-26.503, 7.3378) ccw
  line L8 (-26.9387, 2.3568) -> (-89.1024, 7.7954)
  arc A27 (-98.0342, 19.7304) -> (-89.1024, 7.7954) centre (-88.2308, 17.7574) ccw
  arc A28 (-83.2722, 55.3691) -> (-98.0342, 19.7304) centre (0, 0) ccw
  arc A29 (-68.5171, 57.4927) -> (-83.2722, 55.3691) centre (-74.945, 49.8322) ccw
  line L9 (-68.5171, 57.4927) -> (-20.7151, 17.382)
  arc A30 (-19.5783, 11.0878) -> (-20.7151, 17.382) centre (-23.929, 13.5518) ccw
  arc A31 (-19.5783, 11.0878) -> (-21.6842, 6.0037) centre (0, 0) ccw
  line L10 (-2.3568, -26.9387) -> (-7.7954, -89.1024)
  arc A32 (-19.7304, -98.0342) -> (-7.7954, -89.1024) centre (-17.7574, -88.2308) ccw
  arc A33 (-55.3691, -83.2722) -> (-19.7304, -98.0342) centre (0, 0) ccw
  arc A34 (-57.4927, -68.5171) -> (-55.3691, -83.2722) centre (-49.8322, -74.945) ccw
  line L11 (-57.4927, -68.5171) -> (-17.382, -20.7151)
  arc A35 (-11.0878, -19.5783) -> (-17.382, -20.7151) centre (-13.5518, -23.929) ccw
  arc A36 (-11.0878, -19.5783) -> (-6.0037, -21.6842) centre (0, 0) ccw
  arc A37 (-2.3568, -26.9387) -> (-6.0037, -21.6842) centre (-7.3378, -26.503) ccw
  arc A38 (-6.0037, 21.6842) -> (-2.3568, 26.9387) centre (-7.3378, 26.503) ccw
  arc A39 (-6.0037, 21.6842) -> (-11.0878, 19.5783) centre (0, 0) ccw
  arc A40 (-17.382, 20.7151) -> (-11.0878, 19.5783) centre (-13.5518, 23.929) ccw
  line L12 (-17.382, 20.7151) -> (-57.4927, 68.5171)
  arc A41 (-55.3691, 83.2722) -> (-57.4927, 68.5171) centre (-49.8322, 74.945) ccw
  arc A42 (-19.7304, 98.0342) -> (-55.3691, 83.2722) centre (0, 0) ccw
  arc A43 (-7.7954, 89.1024) -> (-19.7304, 98.0342) centre (-17.7574, 88.2308) ccw
  line L13 (-7.7954, 89.1024) -> (-2.3568, 26.9387)
  line L14 (-20.7151, -17.382) -> (-68.5171, -57.4927)
  arc A44 (-83.2722, -55.3691) -> (-68.5171, -57.4927) centre (-74.945, -49.8322) ccw
  arc A45 (-98.0342, -19.7304) -> (-83.2722, -55.3691) centre (0, 0) ccw
  arc A46 (-89.1024, -7.7954) -> (-98.0342, -19.7304) centre (-88.2308, -17.7574) ccw
  line L15 (-89.1024, -7.7954) -> (-26.9387, -2.3568)
  arc A47 (-21.6842, -6.0037) -> (-26.9387, -2.3568) centre (-26.503, -7.3378) ccw
  arc A48 (-21.6842, -6.0037) -> (-19.5783, -11.0878) centre (0, 0) ccw
  arc A49 (-20.7151, -17.382) -> (-19.5783, -11.0878) centre (-23.929, -13.5518) ccw
  circle A50 centre (0, 0) radius 110
  circle A51 centre (0, 0) radius 13
  dimension "d251" = 26
  constraint concentric A3 A51
  measures "d251" diameter of A51
extrude "Extrude3'''" cut sketch "Sketch2 (8)" against normal blind 5 contours A51 bodies 1 in component "Wheel"
sketch "Sketch10" plane through (0, 8, 0) normal (0, 1, 0) x (-1, 0, 0) in component "Board"
  line L0 (-150, 17.5) -> (-150, -17.5)
  line L1 (-150, -17.5) -> (-140, -17.5)
  line L2 (-140, -17.5) -> (-140, 17.5)
  line L3 (-140, 17.5) -> (-150, 17.5)
  line L4 (-150, -7.5) -> (-140, -7.5)
  line L5 (-140, -7.5) -> (-140, 7.5)
  line L6 (-140, 7.5) -> (-150, 7.5)
  line L7 (-150, 7.5) -> (-150, -7.5)
  line L8 (-150, -7.5) -> (-140, 7.5) construction
  line L9 (-140, -7.5) -> (-150, 7.5) construction
  line L10 (0, 20) -> (0, 2.5)
  line L11 (140, 7.5) -> (150, 7.5)
  line L12 (150, 7.5) -> (150, -7.5)
  line L13 (150, -7.5) -> (140, -7.5)
  line L14 (140, -7.5) -> (140, 7.5)
  point P0 (-145, 0)
  dimension "d265" = 10
  dimension "d266" = 15
  constraint horizontal L4
  constraint perpendicular L4 L5
  constraint parallel L4 L6
  constraint parallel L5 L7
  constraint coincident L8 P0
  constraint coincident L9 P0
  constraint symmetric L4.start L10 L12.end
  constraint symmetric L4.end L10 L13.end
  constraint symmetric L5.end L10 L11.start
  constraint symmetric L6.end L10 L11.end
  measures "d265" distance of L5.end L6.end
  measures "d266" distance of L4.end L5.end
extrude "Extrude6" cut sketch "Sketch10" along normal blind 5 contours L0 L2 L4 L5 L6 L7 | L11 L12 L13 L14 bodies 4 in component "Board"
sketch "Sketch11" plane through (0, 8, 0) normal (0, 1, 0) x (-1, 0, 0) in component "Board"
  line L0 (-150, 17.5) -> (-150, -17.5)
  line L1 (-150, -17.5) -> (-140, -17.5)
  line L2 (-140, -17.5) -> (-140, 17.5)
  line L3 (-140, 17.5) -> (-150, 17.5)
  line L4 (-150, -7.5) -> (-140, -7.5)
  line L5 (-140, -7.5) -> (-140, 7.5)
  line L6 (-140, 7.5) -> (-150, 7.5)
  line L7 (-150, 7.5) -> (-150, -7.5)
  line L8 (-150, -7.5) -> (-140, 7.5) construction
  line L9 (-140, -7.5) -> (-150, 7.5) construction
  line L10 (0, 20) -> (0, 2.5)
  line L11 (140, 7.5) -> (150, 7.5)
  line L12 (140, -7.5) -> (140, 7.5)
  line L13 (150, 7.5) -> (150, -7.5)
  line L14 (150, -7.5) -> (140, -7.5)
  point P0 (-145, 0)
  dimension "d269" = 10
  dimension "d270" = 15
  constraint horizontal L4
  constraint perpendicular L4 L5
  constraint parallel L4 L6
  constraint parallel L5 L7
  constraint coincident L8 P0
  constraint coincident L9 P0
  constraint symmetric L4.start L10 L13.end
  constraint symmetric L4.end L10 L12.start
  constraint symmetric L5.end L10 L11.start
  constraint symmetric L6.end L10 L11.end
  measures "d269" distance of L5.end L6.end
  measures "d270" distance of L4.end L5.end
extrude "Extrude7" add sketch "Sketch11" along normal blind 5 contours L0 L2 L4 L5 L6 L7 | L11 L12 L13 L14 bodies 6 7 in component "Board"